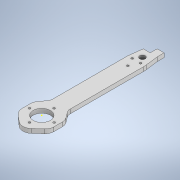
# Autodesk Inventor part: mod arms
Saved by Autodesk Inventor 2020 (Build 240168000, 168)
## iProperties
Created: 2021-11-30
Part Number: mod arms
Material: Generic
Document SubType Name: Modeling
Designer: Steven
Density: 1 g/cm^3
Appearance: Default
Author: Steven
Autodesk Inventor part; units mm, degrees
ref_plane "YZ Plane" through (0, 0, 0) normal (1, 0, 0) x (0, 1, 0)
ref_plane "XZ Plane" through (0, 0, 0) normal (0, 1, 0) x (-1, 0, 0)
ref_plane "XY Plane" through (0, 0, 0) normal (0, 0, 1) x (1, 0, 0)
sketch "Sketch1" plane through (0, 0, 0) normal (0, 1, 0) x (-1, 0, 0)
  arc A0 (4.5962, 6.7175) -> (6.7175, 4.5962) centre (5.6569, 5.6569) ccw
  line L0 (5.6569, 7.7782) -> (4.5962, 6.7175)
  arc A1 (7.7782, 5.6569) -> (5.6569, 7.7782) centre (6.7175, 6.7175) ccw
  line L1 (6.7175, 4.5962) -> (7.7782, 5.6569)
  circle A2 centre (0, 0) radius 3
  circle A3 centre (0, -124.0736) radius 1.5
  circle A4 centre (0, -145.2868) radius 4
  arc A5 (-4.5962, -6.7175) -> (-6.7175, -4.5962) centre (-5.6569, -5.6569) ccw
  line L2 (-5.6569, -7.7782) -> (-4.5962, -6.7175)
  arc A6 (-7.7782, -5.6569) -> (-5.6569, -7.7782) centre (-6.7175, -6.7175) ccw
  line L3 (-6.7175, -4.5962) -> (-7.7782, -5.6569)
  line L4 (-20, 5.4953) -> (-20, -6.6667)
  arc A7 (-20, -6.6667) -> (-18, -12.6667) centre (-10, -6.6667) ccw
  line L5 (-18, -12.6667) -> (-14.5, -17.3333)
  arc A8 (-12.5, -23.3333) -> (-14.5, -17.3333) centre (-22.5, -23.3333) ccw
  line L6 (-12.5, -23.3333) -> (-12.5, -134.321)
  arc A9 (-12.5, -134.321) -> (-12.2297, -138.6622) centre (22.5, -134.321) ccw
  line L7 (-12.2297, -138.6622) -> (-10, -156.5)
  line L8 (-10, -156.5) -> (-10, -166.5)
  line L9 (-10, -166.5) -> (0, -166.5)
  line L10 (0, -166.5) -> (0, -156.5)
  line L11 (0, -156.5) -> (10, -156.5)
  line L12 (10, -156.5) -> (12.2297, -138.6622)
  arc A10 (12.2297, -138.6622) -> (12.5, -134.321) centre (-22.5, -134.321) ccw
  line L13 (12.5, -134.321) -> (12.5, -23.3333)
  arc A11 (14.5, -17.3333) -> (12.5, -23.3333) centre (22.5, -23.3333) ccw
  line L14 (14.5, -17.3333) -> (18, -12.6667)
  arc A12 (18, -12.6667) -> (20, -6.6667) centre (10, -6.6667) ccw
  line L15 (20, -6.6667) -> (20, 5.4953)
  arc A13 (20, 5.4953) -> (16.6262, 12.9849) centre (10, 5.4953) ccw
  line L16 (16.6262, 12.9849) -> (6.6262, 21.8321)
  arc A14 (6.6262, 21.8321) -> (-6.6262, 21.8321) centre (0, 14.3426) ccw
  line L17 (-6.6262, 21.8321) -> (-16.6262, 12.9849)
  arc A15 (-16.6262, 12.9849) -> (-20, 5.4953) centre (-10, 5.4953) ccw
  arc A16 (-6.7175, 4.5962) -> (-4.5962, 6.7175) centre (-5.6569, 5.6569) ccw
  line L18 (-7.7782, 5.6569) -> (-6.7175, 4.5962)
  arc A17 (-5.6569, 7.7782) -> (-7.7782, 5.6569) centre (-6.7175, 6.7175) ccw
  line L19 (-4.5962, 6.7175) -> (-5.6569, 7.7782)
  arc A18 (6.7175, -4.5962) -> (4.5962, -6.7175) centre (5.6569, -5.6569) ccw
  line L20 (7.7782, -5.6569) -> (6.7175, -4.5962)
  arc A19 (5.6569, -7.7782) -> (7.7782, -5.6569) centre (6.7175, -6.7175) ccw
  line L21 (4.5962, -6.7175) -> (5.6569, -7.7782)
  circle A20 centre (6, -136.5) radius 1.5
  circle A21 centre (-6, -136.5) radius 1.5
  point P0 (18, -12.6667)
  point P1 (16.6262, 12.9849)
  point P2 (6.6262, 21.8321)
  point P3 (-6.6262, 21.8321)
  point P4 (-16.6262, 12.9849)
  point P5 (-18, -12.6667)
  point P6 (-14.5, -17.3333)
  point P7 (-12.5, -23.3333)
  point P8 (-12.5, -134.321)
  point P9 (-12.2297, -138.6622)
  point P10 (12.2297, -138.6622)
  point P11 (12.5, -134.321)
  point P12 (12.5, -23.3333)
  point P13 (14.5, -17.3333)
  point P14 (-6.7175, -4.5962)
  point P15 (-4.5962, -6.7175)
  point P16 (-5.6569, -7.7782)
  point P17 (-7.7782, -5.6569)
  point P18 (7.7782, 5.6569)
  point P19 (6.7175, 4.5962)
  point P20 (4.5962, 6.7175)
  point P21 (5.6569, 7.7782)
  point P22 (-5.6569, 7.7782)
  point P23 (-4.5962, 6.7175)
  point P24 (-6.7175, 4.5962)
  point P25 (-7.7782, 5.6569)
  point P26 (6.7175, -4.5962)
  point P27 (7.7782, -5.6569)
  point P28 (5.6569, -7.7782)
  point P29 (4.5962, -6.7175)
  constraints: 44 end point, 34 point on circle, 22 centre point
extrude "Extrusion1" add sketch "Sketch1" along normal blind 6
sketch "Sketch2" plane through (0, 6, 0) normal (0, 1, 0) x (1, 0, 0)
  line L0 (20, -5.4953) -> (20, 6.6667) projected
  arc A0 (20, 6.6667) -> (18, 12.6667) centre (10, 6.6667) ccw projected
  line L1 (18, 12.6667) -> (14.5, 17.3333) projected
  arc A1 (12.5, 23.3333) -> (14.5, 17.3333) centre (22.5, 23.3333) ccw projected
  line L2 (12.5, 23.3333) -> (12.5, 134.321) projected
  arc A2 (12.5, 134.321) -> (12.2297, 138.6622) centre (-22.5, 134.321) ccw projected
  line L3 (12.2297, 138.6622) -> (10, 156.5) projected
  line L4 (10, 156.5) -> (10, 166.5) projected
  line L5 (10, 166.5) -> (0, 166.5) projected
  line L6 (0, 166.5) -> (0, 156.5) projected
  line L7 (0, 156.5) -> (-10, 156.5) projected
  line L8 (-10, 156.5) -> (-12.2297, 138.6622) projected
  arc A3 (-12.2297, 138.6622) -> (-12.5, 134.321) centre (22.5, 134.321) ccw projected
  line L9 (-12.5, 134.321) -> (-12.5, 23.3333) projected
  arc A4 (-14.5, 17.3333) -> (-12.5, 23.3333) centre (-22.5, 23.3333) ccw projected
  line L10 (-14.5, 17.3333) -> (-18, 12.6667) projected
  arc A5 (-18, 12.6667) -> (-20, 6.6667) centre (-10, 6.6667) ccw projected
  line L11 (-20, 6.6667) -> (-20, -5.4953) projected
  arc A6 (-20, -5.4953) -> (-16.6262, -12.9849) centre (-10, -5.4953) ccw projected
  line L12 (-16.6262, -12.9849) -> (-6.6262, -21.8321) projected
  arc A7 (-6.6262, -21.8321) -> (6.6262, -21.8321) centre (0, -14.3426) ccw projected
  line L13 (6.6262, -21.8321) -> (16.6262, -12.9849) projected
  arc A8 (16.6262, -12.9849) -> (20, -5.4953) centre (10, -5.4953) ccw projected
  circle A9 centre (0, 0) radius 3 projected
  circle A10 centre (0, 145.2868) radius 4 projected
  circle A11 centre (-6, 136.5) radius 1.5 projected
  circle A12 centre (6, 136.5) radius 1.5 projected
  circle A13 centre (0, 124.0736) radius 1.5 projected
  line L14 (7.7782, 5.6569) -> (6.7175, 4.5962) projected
  arc A14 (4.5962, 6.7175) -> (6.7175, 4.5962) centre (5.6569, 5.6569) ccw projected
  line L15 (4.5962, 6.7175) -> (5.6569, 7.7782) projected
  arc A15 (7.7782, 5.6569) -> (5.6569, 7.7782) centre (6.7175, 6.7175) ccw projected
  line L16 (-7.7782, -5.6569) -> (-6.7175, -4.5962) projected
  arc A16 (-4.5962, -6.7175) -> (-6.7175, -4.5962) centre (-5.6569, -5.6569) ccw projected
  line L17 (-4.5962, -6.7175) -> (-5.6569, -7.7782) projected
  arc A17 (-7.7782, -5.6569) -> (-5.6569, -7.7782) centre (-6.7175, -6.7175) ccw projected
  arc A18 (5.6569, -7.7782) -> (7.7782, -5.6569) centre (6.7175, -6.7175) ccw projected
  line L18 (5.6569, -7.7782) -> (4.5962, -6.7175) projected
  arc A19 (6.7175, -4.5962) -> (4.5962, -6.7175) centre (5.6569, -5.6569) ccw projected
  line L19 (6.7175, -4.5962) -> (7.7782, -5.6569) projected
  line L20 (-6.7175, 4.5962) -> (-7.7782, 5.6569) projected
  arc A20 (-5.6569, 7.7782) -> (-7.7782, 5.6569) centre (-6.7175, 6.7175) ccw projected
  line L21 (-5.6569, 7.7782) -> (-4.5962, 6.7175) projected
  arc A21 (-6.7175, 4.5962) -> (-4.5962, 6.7175) centre (-5.6569, 5.6569) ccw projected
  line L22 (18.6141, -15.2318) -> (8.6141, -24.079)
  arc A22 (-8.6141, -24.079) -> (8.6141, -24.079) centre (0, -14.3426) ccw
  line L23 (-8.6141, -24.079) -> (-18.6141, -15.2318)
  arc A23 (-23, -5.4953) -> (-18.6141, -15.2318) centre (-10, -5.4953) ccw
  line L24 (-23, -5.4953) -> (-23, 6.6667)
  arc A24 (-20.4, 14.4667) -> (-23, 6.6667) centre (-10, 6.6667) ccw
  line L25 (-20.4, 14.4667) -> (-12.5, 25)
  line L26 (-15.5, 23.3333) -> (-15.5, 134.321)
  arc A25 (-15.2066, 139.0343) -> (-15.5, 134.321) centre (22.5, 134.321) ccw
  line L27 (-15.2066, 139.0343) -> (-12.6483, 159.5)
  line L28 (-12.6483, 159.5) -> (-3, 159.5)
  line L29 (-3, 159.5) -> (-3, 169.5)
  line L30 (-3, 169.5) -> (13, 169.5)
  line L31 (13, 169.5) -> (13, 156.6868)
  line L32 (13, 156.6868) -> (15.2066, 139.0343)
  arc A26 (15.5, 134.321) -> (15.2066, 139.0343) centre (-22.5, 134.321) ccw
  line L33 (15.5, 134.321) -> (15.5, 23.3333)
  line L34 (12.5, 25) -> (20.4, 14.4667)
  arc A27 (23, 6.6667) -> (20.4, 14.4667) centre (10, 6.6667) ccw
  line L35 (23, 6.6667) -> (23, -5.4953)
  arc A28 (18.6141, -15.2318) -> (23, -5.4953) centre (10, -5.4953) ccw
  dimension "d2" = 3
  constraints: 28 end point, 14 point on circle, 7 centre point, 2 point on line, 16 other
  measures "d2" distance between parallel lines of L13 L22
extrude "Extrusion2" add sketch "Sketch2" against normal blind 6 contours L0 A0 L1 A1 L2 L34 A27 L35 A28 L22 A22 L23 A23 L24 A24 L25 L9 A4 L10 A5 L11 A6 L12 A7 L13 A8
sketch "Sketch3" plane through (0, 6, 0) normal (0, 1, 0) x (1, 0, 0)
  line L0 (12.5, 25) -> (12.5, 134.321) projected
  arc A0 (12.5, 134.321) -> (12.2297, 138.6622) centre (-22.5, 134.321) ccw projected
  line L1 (12.2297, 138.6622) -> (10, 156.5) projected
  line L2 (10, 156.5) -> (10, 166.5) projected
  line L3 (10, 166.5) -> (0, 166.5) projected
  line L4 (0, 166.5) -> (0, 156.5) projected
  line L5 (0, 156.5) -> (-10, 156.5) projected
  line L6 (-10, 156.5) -> (-12.2297, 138.6622) projected
  arc A1 (-12.2297, 138.6622) -> (-12.5, 134.321) centre (22.5, 134.321) ccw projected
  line L7 (-12.5, 134.321) -> (-12.5, 25) projected
  circle A2 centre (0, 0) radius 3 projected
  circle A3 centre (0, 145.2868) radius 4 projected
  circle A4 centre (-6, 136.5) radius 1.5 projected
  circle A5 centre (6, 136.5) radius 1.5 projected
  circle A6 centre (0, 124.0736) radius 1.5 projected
  line L8 (7.7782, 5.6569) -> (6.7175, 4.5962) projected
  arc A7 (4.5962, 6.7175) -> (6.7175, 4.5962) centre (5.6569, 5.6569) ccw projected
  line L9 (4.5962, 6.7175) -> (5.6569, 7.7782) projected
  arc A8 (7.7782, 5.6569) -> (5.6569, 7.7782) centre (6.7175, 6.7175) ccw projected
  line L10 (-7.7782, -5.6569) -> (-6.7175, -4.5962) projected
  arc A9 (-4.5962, -6.7175) -> (-6.7175, -4.5962) centre (-5.6569, -5.6569) ccw projected
  line L11 (-4.5962, -6.7175) -> (-5.6569, -7.7782) projected
  arc A10 (-7.7782, -5.6569) -> (-5.6569, -7.7782) centre (-6.7175, -6.7175) ccw projected
  arc A11 (5.6569, -7.7782) -> (7.7782, -5.6569) centre (6.7175, -6.7175) ccw projected
  line L12 (5.6569, -7.7782) -> (4.5962, -6.7175) projected
  arc A12 (6.7175, -4.5962) -> (4.5962, -6.7175) centre (5.6569, -5.6569) ccw projected
  line L13 (6.7175, -4.5962) -> (7.7782, -5.6569) projected
  line L14 (-6.7175, 4.5962) -> (-7.7782, 5.6569) projected
  arc A13 (-5.6569, 7.7782) -> (-7.7782, 5.6569) centre (-6.7175, 6.7175) ccw projected
  line L15 (-5.6569, 7.7782) -> (-4.5962, 6.7175) projected
  arc A14 (-6.7175, 4.5962) -> (-4.5962, 6.7175) centre (-5.6569, 5.6569) ccw projected
  line L16 (-12.5, 25) -> (-20.4, 14.4667) projected
  arc A15 (-20.4, 14.4667) -> (-23, 6.6667) centre (-10, 6.6667) ccw projected
  line L17 (-23, 6.6667) -> (-23, -5.4953) projected
  arc A16 (-23, -5.4953) -> (-18.6141, -15.2318) centre (-10, -5.4953) ccw projected
  line L18 (-18.6141, -15.2318) -> (-8.6141, -24.079) projected
  arc A17 (-8.6141, -24.079) -> (8.6141, -24.079) centre (0, -14.3426) ccw projected
  line L19 (8.6141, -24.079) -> (18.6141, -15.2318) projected
  arc A18 (18.6141, -15.2318) -> (23, -5.4953) centre (10, -5.4953) ccw projected
  line L20 (23, -5.4953) -> (23, 6.6667) projected
  arc A19 (23, 6.6667) -> (20.4, 14.4667) centre (10, 6.6667) ccw projected
  line L21 (20.4, 14.4667) -> (12.5, 25) projected
  circle A20 centre (-6.7175, -6.7175) radius 3 construction
  line L22 (0, 0) -> (-8.8388, -8.8388) construction
  circle A21 centre (0, 0) radius 12.5
  dimension "d8" = 6
  constraints: 2 coincident, 2 end point, 6 other
fillet "Fillet1" radius 10 2 edges at (12.5, 3, -25) (-12.5, 3, -25)
extrude "Extrusion3" cut sketch "Sketch3" against normal blind 6 contours A21
sketch "Sketch4" plane through (0, 6, 0) normal (0, 1, 0) x (1, 0, 0)
  circle A0 centre (0, 0) radius 12.5 construction
  circle A1 centre (0, 0) radius 12.5 construction
  line L0 (12.5, 0) -> (23, 0) construction
  line L1 (23, -5.4953) -> (23, 6.6667) construction
  circle A2 centre (0, 0) radius 17.75 construction
  line L2 (0, -12.5) -> (0, -17.75) construction
  line L3 (-12.5, 0) -> (-17.75, 0) construction
  line L4 (0, 12.5) -> (0, 17.75) construction
  circle A3 centre (17.75, 0) radius 1.5
  circle A4 centre (0, 17.75) radius 1.5
  circle A5 centre (-17.75, 0) radius 1.5
  circle A6 centre (0, -17.75) radius 1.5
  dimension "d11" = 3
  dimension "d14" = 360
  constraints: 8 end point, 8 point on circle, 6 centre point, 3 point on line, 2 coincident, 1 horizontal, 1 midpoint, 1 perpendicular, 1 vertical, 9 other
  measures "d11" diameter of A3
extrude "Extrusion4" cut sketch "Sketch4" against normal up to next
sketch "Sketch5" plane through (0, 6, 0) normal (0, 1, 0) x (1, 0, 0)
  point P0 (0, 0)
body "Solid1"
